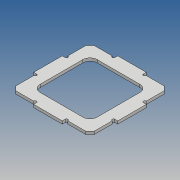
# Autodesk Inventor part: refuerzo interior
Saved by Autodesk Inventor 2017 (Build 210142000, 142)
## iProperties
Part Number: refuerzo interior
Material: Genérico
Document SubType Name: Modeling
Designer: Leo
Density: 1 g/cm^3
Appearance: Valor por defecto
Author: Leo
Autodesk Inventor part; units mm, degrees
ref_plane "YZ Plane" through (0, 0, 0) normal (1, 0, 0) x (0, 1, 0)
ref_plane "XZ Plane" through (0, 0, 0) normal (0, 1, 0) x (-1, 0, 0)
ref_plane "XY Plane" through (0, 0, 0) normal (0, 0, 1) x (1, 0, 0)
sketch "Boceto1" plane through (0, 0, 0) normal (0, 0, 1) x (1, 0, 0)
  line L0 (0, 82.4534) -> (0, -82.4534) construction
  line L1 (-81.8976, 0) -> (81.8976, 0) construction
  line L2 (55, 49) -> (55, 24)
  arc A0 (55, 24) -> (55, 20) centre (55, 22) ccw
  line L3 (55, 20) -> (59, 20)
  line L4 (59, 20) -> (59, -20)
  line L5 (59, -20) -> (55, -20)
  arc A1 (55, -20) -> (55, -24) centre (55, -22) ccw
  line L6 (55, -24) -> (55, -49)
  line L7 (-55, 49) -> (-55, 24)
  arc A2 (-55, 20) -> (-55, 24) centre (-55, 22) ccw
  line L8 (-55, 20) -> (-59, 20)
  line L9 (-59, 20) -> (-59, -20)
  line L10 (-59, -20) -> (-55, -20)
  arc A3 (-55, -24) -> (-55, -20) centre (-55, -22) ccw
  line L11 (-55, -24) -> (-55, -49)
  line L12 (-49, 55) -> (-24, 55)
  line L13 (24, 55) -> (49, 55)
  line L14 (-49, -55) -> (-24, -55)
  line L15 (24, -55) -> (49, -55)
  arc A4 (-24, 55) -> (-20, 55) centre (-22, 55) ccw
  line L16 (-20, 55) -> (-20, 59)
  line L17 (-20, 59) -> (20, 59)
  line L18 (20, 59) -> (20, 55)
  arc A5 (20, 55) -> (24, 55) centre (22, 55) ccw
  arc A6 (-20, -55) -> (-24, -55) centre (-22, -55) ccw
  line L19 (-20, -55) -> (-20, -59)
  line L20 (-20, -59) -> (20, -59)
  line L21 (20, -59) -> (20, -55)
  arc A7 (24, -55) -> (20, -55) centre (22, -55) ccw
  line L22 (-55, 49) -> (-49, 55)
  line L23 (55, 49) -> (49, 55)
  line L24 (55, -49) -> (49, -55)
  line L25 (-49, -55) -> (-55, -49)
  line L26 (-40, 30) -> (-40, -30)
  arc A8 (-40, -30) -> (-30, -40) centre (-30, -30) ccw
  line L27 (-30, -40) -> (30, -40)
  arc A9 (30, -40) -> (40, -30) centre (30, -30) ccw
  line L28 (40, -30) -> (40, 30)
  arc A10 (40, 30) -> (30, 40) centre (30, 30) ccw
  line L29 (30, 40) -> (-30, 40)
  arc A11 (-30, 40) -> (-40, 30) centre (-30, 30) ccw
  point P0 (0, 0)
  point P1 (0, 0)
  point P2 (55, 55)
  point P3 (55, -55)
  point P4 (-55, 55)
  point P5 (-55, -55)
  point P6 (55, -55)
  point P7 (-59, 0)
  point P8 (55, -55)
  point P9 (-40, 0)
  point P10 (0, 40)
  dimension "d0" = 110
  dimension "d1" = 40
  dimension "d2" = 2
  dimension "d3" = 110
  dimension "d7" = 4
  dimension "d8" = 6
  dimension "d9" = 6
  dimension "d10" = 6
  dimension "d11" = 6
  dimension "d12" = 6
  dimension "d13" = 6
  dimension "d14" = 6
  dimension "d15" = 6
  dimension "d16" = 15
  dimension "d17" = 10
  constraints: 60 end point, 24 point on circle, 22 point on line, 20 symmetric about line, 12 centre point, 12 tangent, 7 perpendicular, 6 equal radius, 5 midpoint, 5 vertical, 4 equal length, 3 horizontal, 1 coincident, 1 collinear, 4 other
  measures "d0" distance between parallel lines of L2 L7
  measures "d1" distance of L8.end L9.end
  measures "d2" radius of A2
  measures "d3" distance between parallel lines of L12 L14
  measures "d7" distance between parallel lines of L7 L9
  measures "d8" distance of L7.start point (-55, 55)
  measures "d9" distance of L12.start point (-55, 55)
  measures "d10" distance of L2.start point (55, 55)
  measures "d11" distance of L13.end point (55, 55)
  measures "d12" distance of L6.end point (55, -55)
  measures "d13" distance of L15.end point (55, -55)
  measures "d14" distance of L14.start point (-55, -55)
  measures "d15" distance of L11.end point (-55, -55)
  measures "d16" distance between parallel lines of L28 L2
  measures "d17" radius of A11
extrude "Extrusión1" add sketch "Boceto1" along normal mid plane 4
equation "\"d9\" = d8"
equation "\"d10\" = d8"
equation "\"d11\" = d10"
equation "\"d12\" = d8"
equation "\"d13\" = d12"
equation "\"d14\" = d8"
equation "\"d15\" = d14"
